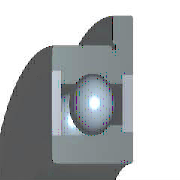
# Autodesk Inventor part: Bearing F 61800-2Z GB/T 7218
Saved by Autodesk Inventor 2024.3 (Build 283343000, 343)
## iProperties
Created: 2023-01-19
Part Number: Bearing F 61800-2Z GB/T 7218
Material: Steel, Mild
Description: Rolling bearings Miniature radial ball bearings with flanged outer ring Boundary dimensions
Document SubType Name: Modeling
Standard: GB/T 7218-2013
Designer: Niler
Standard Revision: 2013
Standards Organization: GB
Language: en-US
Size Designation: F 61800-2Z
Categories: <MemberInstance><Categories><Category DisplayName="Shaft Parts" InternalName="7f7aeb1f-a693-4053-b835-cee3144e0d98" Mnemonic="SHFT"><Category DisplayName="Bearings" InternalName="242d30a3-7172-44e6-a363-b0a3d8f1b556" Mnemonic="BRNG"><CategoryParameter DisplayName="Width" InternalName="25fc5f6e-338b-4801-b5ed-8959743e396e" Mnemonic="wdth"/><CategoryParameter DisplayName="Size Designation" InternalName="2c4e891a-c8f4-49ed-a5c1-5131476c6feb" Mnemonic="sizedes"/><CategoryParameter DisplayName="Basic Dynamic Load Rating" InternalName="440972dd-7009-4861-bd45-69ffbb461423" Mnemonic="bdynlrat"/><CategoryParameter DisplayName="Shaft Diameter" InternalName="91302473-2833-4451-a660-c5d4a8d6a031" Mnemonic="shaftdia"/><CategoryParameter DisplayName="Touch Angle" InternalName="aa21a452-7974-4a55-b5cf-1c2972de2aea" Mnemonic="TouchAngle"/><CategoryParameter DisplayName="Outer Diameter" InternalName="d441686c-04bd-4681-b674-94fbc173ec23" Mnemonic="outdia"/><Category DisplayName="Ball Bearings" InternalName="9b553946-0899-4a5e-a403-c1d9295e77c1" Mnemonic="BALLBEAR"><CategoryParameter DisplayName="Radial Dynamic Load Factor when Fa/Fr &lt;= e" InternalName="051e59b3-bd55-4dad-8b07-38b5cb912881" Mnemonic="raddynfc1"/><CategoryParameter DisplayName="Basic Static Load Rating" InternalName="0f13fbbf-c511-4d43-b4c7-197b47424baf" Mnemonic="bstatlrat"/><CategoryParameter DisplayName="Exponent for Determining Life" InternalName="3029e2ef-9460-4be8-bdfd-dfe61437473d" Mnemonic="lifeexp"/><CategoryParameter DisplayName="Friction Factor" InternalName="3086b0f2-3d69-46ff-8a75-fe12e395bb47" Mnemonic="fricfct"/><CategoryParameter DisplayName="Min. Shaft Diameter" InternalName="4a5be9bc-ad86-4bf2-8167-102dad5d3e27" Mnemonic="minshaftdia"/><CategoryParameter DisplayName="Axial Dynamic Load Factor when Fa/Fr &gt; e" InternalName="4b6ff741-5956-4a40-80f5-34eb9259f88c" Mnemonic="axdynfc2"/><CategoryParameter DisplayName="Limiting Speed Lubrication Grease" InternalName="5237843b-2c8d-46d3-8227-f3e9dd85a12e" Mnemonic="lubgrsp"/><CategoryParameter DisplayName="Limiting Speed Oil" InternalName="60628548-8907-44dc-8e09-603d72f5766f" Mnemonic="oilspd"/><CategoryParameter DisplayName="Axial Static Load Factor" InternalName="74dbf5e2-8362-409a-802f-3c2235668d99" Mnemonic="axdynfc0"/><CategoryParameter DisplayName="Mass" InternalName="7b80f85c-da81-4dea-b8db-d7c689da91b2" Mnemonic="mass"/><CategoryParameter DisplayName="Radius" InternalName="83352640-dfae-4cba-bc9f-11ecbfb0001c" Mnemonic="rad"/><CategoryParameter DisplayName="Radial Static Load Factor" InternalName="83ce084d-c51e-4598-a871-e8e1e34b26ee" Mnemonic="raddynfc0"/><CategoryParameter DisplayName="Axial Dynamic Load Factor when Fa/Fr &lt;= e" InternalName="ae45a7db-08df-4411-99a8-2f035015bff9" Mnemonic="axdynfc1"/><CategoryParameter DisplayName="Max. Hub Step Diameter" InternalName="b5cf89e0-ca87-439c-b08c-a25e2999ab06" Mnemonic="maxhubdia"/><CategoryParameter DisplayName="Limiting Value for Factor Determination" InternalName="be0ce6fc-cad4-4218-b484-c34dd2571812" Mnemonic="limvalfac"/><CategoryParameter DisplayName="Radial Dynamic Load Factor when Fa/Fr &gt; e" InternalName="e513bdb7-139f-4b3c-af32-49e0ba1226b9" Mnemonic="raddynfc2"/><CategoryParameter DisplayName="Max. Step Fillet Radius" InternalName="f6ce6695-cf2c-4ec9-8d20-66671e0e35a4" Mnemonic="maxstprad"/><Category DisplayName="Angular Contact Ball Bearings" InternalName="0b8e5904-7bca-4d33-b75b-fd5460312790" Mnemonic="BBACBB"/></Category></Category></Category><Category DisplayName="DataType" InternalName="23b78d0f-2648-40c6-8793-ca6db495c9e8" Mnemonic="DATATYPE"><CategoryParameter DisplayName="DisplayName" InternalName="05415f3d-3907-474b-a020-eb9d644f4cf3" Mnemonic="DISPLAYNAME"/><CategoryParameter DisplayName="Standard" InternalName="0c0a119c-1e12-4c84-803f-101930972f5e" Mnemonic="STANDARD"/><CategoryParameter DisplayName="Description" InternalName="13903e3d-64b1-4950-80da-f627842ea37f" Mnemonic="DESCRIPTION"/><CategoryParameter DisplayName="Designation" InternalName="2675968c-4ce5-49e0-a4f5-552d29089031" Mnemonic="DESIGNATION"/><CategoryParameter DisplayName="Default Row" InternalName="2af9ec52-faaa-4026-b378-f9fa4afca842" Mnemonic="DEFAULTROW"/><CategoryParameter DisplayName="Folder Name" InternalName="3f06958e-8713-4116-9be7-ed6184ecc97b" Mnemonic="FOLDERNAME"/><CategoryParameter DisplayName="Revision Guid" InternalName="45a75005-10b1-4dfc-8d6d-dfe629f0b93c" Mnemonic="REVISIONGUID"/><CategoryParameter DisplayName="FileName" InternalName="8b46a4cc-9585-4fed-90c3-899f57e09a73" Mnemonic="FILENAME"/><CategoryParameter DisplayName="StdsOrg" InternalName="8f5914e1-4693-403f-8ab5-d37768198c9d" Mnemonic="STDSORG"/><CategoryParameter DisplayName="Family Version" InternalName="914462f6-6e19-4b14-ba84-155b9680b1d0" Mnemonic="FAMILYREVISION"/><CategoryParameter DisplayName="Standard Revision" InternalName="91d5a463-65c2-4fde-b823-3b7fea5e8e17" Mnemonic="STANDARDREVISION"/><CategoryParameter DisplayName="Member Revision" InternalName="a65d44b9-392f-4f4f-857b-e4b3d54996fe" Mnemonic="MEMBERREVISION"/><CategoryParameter DisplayName="ClipFormat" InternalName="bc51e27b-3422-4e78-93ef-cec197ddf230" Mnemonic="CLIPFORMAT"/><CategoryParameter DisplayName="Manufacturer" InternalName="cd6c7a72-a28a-4e50-99a9-2c7f4e13e5ad" Mnemonic="MANUFACTURER"/><CategoryParameter DisplayName="InternalName" InternalName="cf1d0246-76d9-4b4a-8305-fa0409afb5c1" Mnemonic="INTERNALNAME"/><CategoryParameter DisplayName="IsMetric" InternalName="e2385c5b-1ea4-4823-96a8-8de651266ec3" Mnemonic="ISMETRIC"/><Category DisplayName="Part" InternalName="c0e0b642-3bcb-4cc8-9e80-f96d35c4afa4" Mnemonic="PART"><CategoryParameter DisplayName="Part Number" InternalName="016b6077-bfbe-49bd-92c9-d8d59c39c941" Mnemonic="PARTNUMBER"/><CategoryParameter DisplayName="Stock Number" InternalName="4dba7c1c-e26c-444e-836c-b08b433409a8" Mnemonic="STOCKNUMBER"/><CategoryParameter DisplayName="Material Key" InternalName="5c9a8adb-dd2b-4535-b97f-0a94a95fe41f" Mnemonic="MATERIALKEY"/><CategoryParameter DisplayName="Material" InternalName="818a152a-d3c3-49ca-80ee-df7d91421b8e" Mnemonic="MATERIAL"/></Category></Category><Category DisplayName="LegacyMap" InternalName="cd87c42b-3e48-431e-b5c0-1cbeb14dfe77" Mnemonic="LEGACYMAP"><CategoryParameter DisplayName="unique DA member ID" InternalName="0918ad47-427f-4fed-ae26-24c81c58f590" Mnemonic="DACOOKIE"/><CategoryParameter DisplayName="Merge11 ID" InternalName="0ee8fb18-e2ed-4f39-96f6-1f4b5f50aa71" Mnemonic="MERGE11"/><CategoryParameter DisplayName="unique CC member ID" InternalName="5193edd4-b2b0-4ab4-9d54-de900eee34e0" Mnemonic="CCCOOKIE"/><CategoryParameter DisplayName="Split ID" InternalName="72b5c83c-be7f-45c4-ae51-9160ea6deb26" Mnemonic="SPLIT"/><CategoryParameter DisplayName="MemberID" InternalName="8e5e0294-fc51-4c8f-b3d7-003dc5ed94f6" Mnemonic="MEMBERID"/><CategoryParameter DisplayName="CatalogName" InternalName="d99d1e27-aa94-4de2-af4c-c348882a6f4f" Mnemonic="CATALOGNAME"/><CategoryParameter DisplayName="FamilyNumber" InternalName="e705e1f4-09cb-413e-91f9-551b4188271e" Mnemonic="FAMILYNUMBER"/></Category></Categories><FamilyTemplate Id="br100603_a"><FamilyTemplateParameters><FamilyTemplateParameter ObjectType="kUserParameterObject" ValueType="xs:double" Id="1" ObjectReferenceKey="ANGL"/><FamilyTemplateParameter ObjectType="kUserParameterObject" ValueType="xs:double" Id="2" ObjectReferenceKey="WR"/><FamilyTemplateParameter ObjectType="kUserParameterObject" ValueType="xs:double" Id="3" ObjectReferenceKey="KAB"/><FamilyTemplateParameter ObjectType="kUserParameterObject" ValueType="xs:double" Id="4" ObjectReferenceKey="BC"/><FamilyTemplateParameter ObjectType="kUserParameterObject" ValueType="xs:double" Id="5" ObjectReferenceKey="R1"/><FamilyTemplateParameter ObjectType="kUserParameterObject" ValueType="xs:double" Id="6" ObjectReferenceKey="KR3S"/><FamilyTemplateParameter ObjectType="kUserParameterObject" ValueType="xs:double" Id="7" ObjectReferenceKey="KR1S"/><FamilyTemplateParameter ObjectType="kUserParameterObject" ValueType="xs:double" Id="8" ObjectReferenceKey="KRS"/><FamilyTemplateParameter ObjectType="kUserParameterObject" ValueType="xs:double" Id="9" ObjectReferenceKey="WD"/><FamilyTemplateParameter ObjectType="kUserParameterObject" ValueType="xs:double" Id="10" ObjectReferenceKey="ND1"/><FamilyTemplateParameter ObjectType="kUserParameterObject" ValueType="xs:double" Id="11" ObjectReferenceKey="ND2"/><FamilyTemplateParameter ObjectType="kUserParameterObject" ValueType="xs:double" Id="12" ObjectReferenceKey="ND3"/><FamilyTemplateParameter ObjectType="kUserParameterObject" ValueType="xs:double" Id="13" ObjectReferenceKey="NBR"/><FamilyTemplateParameter ObjectType="kUserParameterObject" ValueType="xs:double" Id="14" ObjectReferenceKey="KB"/><FamilyTemplateParameter ObjectType="kUserParameterObject" ValueType="xs:double" Id="15" ObjectReferenceKey="BI"/><FamilyTemplateParameter ObjectType="kUserParameterObject" ValueType="xs:double" Id="16" ObjectReferenceKey="BC0"/><FamilyTemplateParameter ObjectType="kUserParameterObject" ValueType="xs:double" Id="17" ObjectReferenceKey="BD"/><FamilyTemplateParameter ObjectType="kUserParameterObject" ValueType="xs:double" Id="18" ObjectReferenceKey="NBR1"/><FamilyTemplateParameter ObjectType="kUserParameterObject" ValueType="xs:double" Id="19" ObjectReferenceKey="NBR2"/><FamilyTemplateParameter ObjectType="kUserParameterObject" ValueType="xs:double" Id="20" ObjectReferenceKey="BR"/><FamilyTemplateParameter ObjectType="kUserParameterObject" ValueType="xs:double" Id="21" ObjectReferenceKey="KR2S"/><FamilyTemplateParameter ObjectType="kUserParameterObject" ValueType="xs:double" Id="22" ObjectReferenceKey="SD2"/><FamilyTemplateParameter ObjectType="kPropertyObject" ValueType="xs:string" Id="100" ObjectReferenceKey="{32853F0F-3444-11d1-9E93-0060B03C1CA6}" SubObjectId="52"/><FamilyTemplateParameter ObjectType="kPropertyObject" ValueType="xs:string" Id="105" ObjectReferenceKey="{32853F0F-3444-11d1-9E93-0060B03C1CA6}" SubObjectId="5"/><FamilyTemplateParameter ObjectType="kPartComponentDefinitionObject" ValueType="xs:string" Id="110" SubObjectId="Material"/></FamilyTemplateParameters></FamilyTemplate><CategoryParameterMap><ParamToTemplateMap><ParamToTemplate CategoryParameter="//CategoryParameter[@InternalName='05415f3d-3907-474b-a020-eb9d644f4cf3']" ConstantValue="Rolling bearing GB/T 7218 Type FSN 70000-2Z, F 60000-2Z"/><ParamToTemplate CategoryParameter="//CategoryParameter[@InternalName='cf1d0246-76d9-4b4a-8305-fa0409afb5c1']" ConstantValue="947DF4DE-02FB-40ED-8DA3-00DBCE178834"/><ParamToTemplate CategoryParameter="//CategoryParameter[@InternalName='3f06958e-8713-4116-9be7-ed6184ecc97b']" ConstantValue="GB_T 7218 FSN-2Z"/><ParamToTemplate CategoryParameter="//CategoryParameter[@InternalName='914462f6-6e19-4b14-ba84-155b9680b1d0']" ConstantValue="10"/><ParamToTemplate CategoryParameter="//CategoryParameter[@InternalName='bc51e27b-3422-4e78-93ef-cec197ddf230']" ConstantValue="CF_INVENTOR.STDPARTS"/><ParamToTemplate CategoryParameter="//CategoryParameter[@InternalName='e2385c5b-1ea4-4823-96a8-8de651266ec3']" ConstantValue="true"/><ParamToTemplate CategoryParameter="//CategoryParameter[@InternalName='13903e3d-64b1-4950-80da-f627842ea37f']" ConstantValue="Rolling bearings Miniature radial ball bearings with flanged outer ring Boundary dimensions"/><ParamToTemplate CategoryParameter="//CategoryParameter[@InternalName='8f5914e1-4693-403f-8ab5-d37768198c9d']" ConstantValue="GB"/><ParamToTemplate CategoryParameter="//CategoryParameter[@InternalName='0c0a119c-1e12-4c84-803f-101930972f5e']" ConstantValue="GB/T 7218-2013"/><ParamToTemplate CategoryParameter="//CategoryParameter[@InternalName='cd6c7a72-a28a-4e50-99a9-2c7f4e13e5ad']" TemplateParameter="104"/><ParamToTemplate CategoryParameter="//CategoryParameter[@InternalName='91d5a463-65c2-4fde-b823-3b7fea5e8e17']" ConstantValue="2013"/><ParamToTemplate CategoryParameter="//CategoryParameter[@InternalName='45a75005-10b1-4dfc-8d6d-dfe629f0b93c']" ConstantValue="cb4e30be-e02b-46d3-a2c1-021882e7b820"/><ParamToTemplate CategoryParameter="//CategoryParameter[@InternalName='2af9ec52-faaa-4026-b378-f9fa4afca842']" ConstantValue="10"/><ParamToTemplate CategoryParameter="//CategoryParameter[@InternalName='d99d1e27-aa94-4de2-af4c-c348882a6f4f']" ConstantValue="GB"/><ParamToTemplate CategoryParameter="//CategoryParameter[@InternalName='e705e1f4-09cb-413e-91f9-551b4188271e']" ConstantValue="357"/><ParamToTemplate CategoryParameter="//CategoryParameter[@InternalName='8b46a4cc-9585-4fed-90c3-899f57e09a73']" ConstantValue="Bearing F 61800-2Z GB/T 7218"/><ParamToTemplate CategoryParameter="//CategoryParameter[@InternalName='a65d44b9-392f-4f4f-857b-e4b3d54996fe']" ConstantValue="48C9BFB6-D08E-4D4F-AA2D-D62F0025BB84"/><ParamToTemplate CategoryParameter="//CategoryParameter[@InternalName='2c4e891a-c8f4-49ed-a5c1-5131476c6feb']" ConstantValue="F 61800-2Z"/><ParamToTemplate CategoryParameter="//CategoryParameter[@InternalName='8e5e0294-fc51-4c8f-b3d7-003dc5ed94f6']" ConstantValue="480"/><ParamToTemplate CategoryParameter="//CategoryParameter[@InternalName='d441686c-04bd-4681-b674-94fbc173ec23']" TemplateParameter="17"/><ParamToTemplate CategoryParameter="//CategoryParameter[@InternalName='2675968c-4ce5-49e0-a4f5-552d29089031']" TemplateParameter="100"/><ParamToTemplate CategoryParameter="//CategoryParameter[@InternalName='25fc5f6e-338b-4801-b5ed-8959743e396e']" TemplateParameter="14"/><ParamToTemplate CategoryParameter="//CategoryParameter[@InternalName='83352640-dfae-4cba-bc9f-11ecbfb0001c']" TemplateParameter="8"/><ParamToTemplate CategoryParameter="//CategoryParameter[@InternalName='818a152a-d3c3-49ca-80ee-df7d91421b8e']" TemplateParameter="110"/><ParamToTemplate CategoryParameter="//CategoryParameter[@InternalName='016b6077-bfbe-49bd-92c9-d8d59c39c941']" TemplateParameter="105"/><ParamToTemplate CategoryParameter="//CategoryParameter[@InternalName='91302473-2833-4451-a660-c5d4a8d6a031']" TemplateParameter="9"/></ParamToTemplateMap></CategoryParameterMap></MemberInstance>
Density: 7.85 g/cm^3
Appearance: Semi-Polished
IsCustomPart: 0
Author: Niler
Autodesk Inventor part; units mm, degrees
note: some values were not read from the file. Left out: dimensions or parameters whose unit could not be read.
ref_plane "YZ Plane" through (0, 0, 0) normal (1, 0, 0) x (0, 1, 0)
ref_plane "XZ Plane" through (0, 0, 0) normal (0, 1, 0) x (-1, 0, 0)
sketch "Sketch1" plane through (0, 0, 0) normal (0, 0, 1) x (1, 0, 0)
  line L0 (-0.7, 0) -> (4.2, 0) projected
  line L1 (0, 5) -> (5, 5)
  line L2 (2.5, 6.08) -> (2.5, 8.42)
  circle A0 centre (2.5, 7.25) radius 1.17
  line L3 (3.67, 7.25) -> (1.33, 7.25)
  line L4 (3.4222, 6.53) -> (4.375, 6.53)
  line L5 (3.5, 1.5694) -> (3.5, 1.5694)
  line L6 (3.4222, 7.97) -> (4.375, 7.97)
  line L7 (1.5778, 7.97) -> (0.625, 7.97)
  line L8 (1.35, 7.97) -> (0, 7.97)
  line L9 (0, 9.5) -> (3.899, 9.5)
  line L10 (3.5, 2.4654) -> (3.5, 2.4654)
  line L11 (5, 10.5) -> (4, 10.5)
  line L12 (4, 10.5) -> (4, 9.601)
  line L13 (4, 9.5) -> (4, 9.5) construction
  line L14 (4, 9.601) -> (4.1219, 9.4791)
  line L15 (3.899, 9.5) -> (4.0209, 9.3781)
  arc A1 (4.0209, 9.3781) -> (4.1219, 9.4791) centre (4.0714, 9.4286) ccw
  line L16 (3.899, 9.5) -> (4, 9.5) construction
  line L17 (4, 9.601) -> (4, 9.5) construction
  line L18 (0, 9.5) -> (0, 8.4346)
  line L19 (0, 6.1437) -> (0, 5)
  line L20 (5, 10.5) -> (5, 8.4346)
  line L21 (5, 6.1437) -> (5, 5)
  line L22 (0, 4.3) -> (0, 0.45) projected
  line L23 (4, 9.5) -> (4.1609, 9.3391) construction
  line L24 (5, 6.53) -> (5, 7.97)
  line L25 (4.375, 7.97) -> (4.375, 6.53)
  line L26 (4.375, 6.1437) -> (5, 6.1437)
  line L27 (4.375, 8.4346) -> (5, 8.4346)
  line L28 (4.375, 8.4346) -> (4.375, 7.97)
  line L29 (4.375, 7.97) -> (5, 7.97)
  line L30 (4.375, 6.53) -> (4.375, 6.1437)
  line L31 (4.375, 6.53) -> (5, 6.53)
  line L32 (5, 8.4346) -> (5, 7.97)
  line L33 (5, 6.53) -> (5, 6.1437)
  line L34 (0, 8.4346) -> (0.625, 8.4346)
  line L35 (0.625, 7.97) -> (0.625, 6.1437)
  line L36 (0, 6.1437) -> (0, 7.97)
  line L37 (0.625, 7.97) -> (0, 7.97)
  line L38 (0.625, 6.1437) -> (0, 6.1437)
  line L39 (0.625, 7.97) -> (0.625, 8.4346)
  line L40 (0, 8.4346) -> (0, 7.97)
  line L41 (0, 6.53) -> (0.625, 6.53)
  line L42 (0.625, 6.53) -> (1.5778, 6.53)
  dimension "d3" = 2.34
  dimension "d1" = 0.0714
  dimension "d2" = 45
  dimension "d4" = 10
  dimension "d5" = 14.5
  dimension "d6" = 19
  dimension "d7" = 21
  dimension "d14" = 5
  dimension "d15" = 1
  dimension "d16" = 2.5
  dimension "d19" = 0.1429
  dimension "d20" = 12.2873
  dimension "d21" = 16.8693
  dimension "d22" = 0.625
  dimension "d27" = 0.72
  dimension "d28" = 0.625
  dimension "d29" = 16.8693
  constraints: 82 end point, 14 perpendicular, 12 parallel, 8 collinear, 7 point on line, 2 midpoint, 2 point on circle, 2 tangent, 1 centre point, 1 symmetric about line, 1 vertical alignment, 13 other
  measures "d1" radius of A1
  measures "d2" angle of L12 L13
  measures "d4" diameter of L1 L0
  measures "d5" diameter of point (2.5, 7.25) L0
  measures "d6" diameter of L9 L0
  measures "d7" diameter of L11 L0
  measures "d14" distance between parallel lines of L22 L20
  measures "d15" distance between parallel lines of L20 L12
  measures "d16" distance from line of L22 point (2.5, 7.25)
  measures "d20" diameter of L26 L0
  measures "d21" diameter of L27 L0
  measures "d22" distance between parallel lines of L24 L25
  measures "d27" distance from line of L6 point (2.5, 7.25)
  measures "d28" distance between parallel lines of L22 L35
  measures "d29" diameter of L34 L0
revolve "Body" add sketch "Sketch1" angle 360 about axis through (-10, 0, 0) along (1, 0, 0) contours L19 L38 L35 L42 A0 L4 L30 L26 L21 L1 | L36 L41 L35 L38 | L26 L30 L31 L33 | L40 L34 L39 L8 | L29 L28 L27 L32 | L39 L34 L18 L9 L15 A1 L14 L12 L11 L20 L27 L28 L6 A0 L7
fillet "Fillet1" radius 0.1 2 edges at (5, -10.5, 0) (4, -10.5, 0)
fillet "Fillet1" radius 0.3 1 edges at (0, -9.5, 0)
fillet "Fillet1" radius 0.15 1 edges at (0, -5, 0)
fillet "Fillet1" radius 0.15 1 edges at (5, -5, 0)
revolve "Ball" add sketch "Sketch1" angle 360 about axis through (3.67, 7.25, 0) along (-1, 0, 0) picked at (2.2412, 7.9805) picked at (2.7588, 7.9805) contours A0 L2 L3 | L3 L2 A0
pattern_circular "Balls" count 10 over 360 about axis through (-10, 0, 0) along (1, 0, 0) of "Ball"
revolve "Ring1" add sketch "Sketch1" angle 360 about axis through (-10, 0, 0) along (1, 0, 0) contours L26 L30 L31 L33 | L31 L25 L29 L24 | L29 L28 L27 L32
sketch "Sketch2" plane through (5, 0, 0) normal (1, 0, 0) x (0, 0, -1)
  circle A0 centre (0, 0) radius 10.4 projected
  circle A1 centre (0, 0) radius 8.4346
  circle A2 centre (0, 0) radius 6.1437
  dimension "d23" = 12.2873
  dimension "d24" = 16.8693
  constraints: 2 centre point, 2 coincident, 2 concentric
  measures "d23" diameter of A2
  measures "d24" diameter of A1
extrude "Indent1" cut sketch "Sketch2" against normal blind 0.02 contours A1
revolve "Ring2" add sketch "Sketch1" angle 360 about axis through (-10, 0, 0) along (1, 0, 0) contours L36 L41 L35 L38 | L36 L8 L35 L41 | L40 L34 L39 L8
ref_plane "Work Plane1" through (0, 0, 0) normal (1, 0, 0) x (0, 0, -1)
sketch "Sketch3" plane through (0, 0, 0) normal (1, 0, 0) x (0, 0, -1)
  circle A0 centre (0, 0) radius 8.4346
  circle A1 centre (0, 0) radius 6.1437
  line L0 (-14.7, 0) -> (14.7, 0) projected
  line L1 (0, -14.7) -> (0, 14.7) projected
  dimension "d31" = 16.8693
  dimension "d32" = 12.2873
  constraints: 2 centre point, 2 midpoint, 1 coincident, 1 concentric
  measures "d31" diameter of A0
  measures "d32" diameter of A1
extrude "Indent2" cut sketch "Sketch3" along normal blind 0.02 contours L0 A1 L1 A0 | A0 L1 A1 L0 | L1 A1 L0 A0 | A0 L0 A1 L1
equation "\"d5\" = 0.5 * WD + 0.5 * BD"
equation "\"d16\" = 0.5 * KB"
equation "\"d27\" = -0.08 * WD + 0.08 * BD"
equation "\"d23\" = ND3"
equation "\"d24\" = ND2"
equation "\"d31\" = ND2"
equation "\"d32\" = ND3"
equation "\"d3\" = -0.26 * WD + 0.26 * BD"
equation "\"d1\" = R1"
equation "\"d2\" = ANGL"
equation "\"d4\" = WD"
equation "\"d6\" = BD"
equation "\"d7\" = SD2"
equation "\"d14\" = KB"
equation "\"d15\" = KAB"
equation "\"d19\" = NBR"
equation "\"d20\" = ND3"
equation "\"d21\" = ND2"
equation "\"d22\" = NBR2"
equation "\"d28\" = NBR1"
equation "\"d29\" = ND2"
equation "\"d10\" = KRS"
equation "\"d11\" = KR1S"
equation "\"d12\" = KR2S"
equation "\"d13\" = KR3S"
equation "\"WD\" = 10"
equation "\"BD\" = 19"
equation "\"KB\" = 5"
equation "\"KAB\" = 1"
equation "\"KRS\" = 0.1 * KAB"
equation "\"SD2\" = 21"
equation "\"NBR\" = 0.142857 * KAB"
equation "\"ANGL\" = 45deg"
equation "\"KR1S\" = 0.3"
equation "\"R1\" = 0.0714286 * KAB"
equation "\"NBR1\" = 0.125 * KB"
equation "\"NBR2\" = 0.125 * KB"
equation "\"ND1\" = 0.35045 * WD + 0.72455 * BD"
equation "\"ND2\" = 0.3423 * WD + 0.7077 * BD"
equation "\"ND3\" = 0.6403 * WD + 0.3097 * BD"
equation "\"KR2S\" = KR3S"
equation "\"KR3S\" = 0.15"
equation "\"d30\" = -KB"
equation "\"WR\" = 0.5 * WD"
equation "\"BR\" = 0.5 * BD"
body "Solid1"
